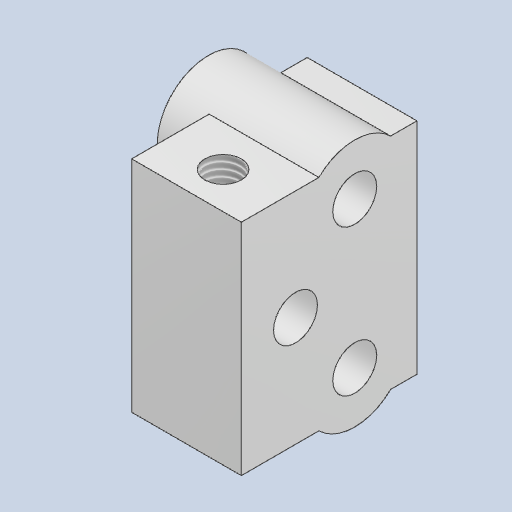
# Autodesk Inventor part: moving_part
Saved by Autodesk Inventor 2024 (Build 280153000, 153)
## iProperties
Created: 2024-09-19
Part Number: moving_part
Material: アルミニウム
Document SubType Name: Modeling
Designer: 1412z
Density: 2.7 g/cm^3
Appearance: サテン
Author: 1412z
Autodesk Inventor part; units mm, degrees
ref_plane "YZ Plane" through (0, 0, 0) normal (1, 0, 0) x (0, 1, 0)
ref_plane "XZ Plane" through (0, 0, 0) normal (0, 1, 0) x (-1, 0, 0)
ref_plane "XY Plane" through (0, 0, 0) normal (0, 0, 1) x (1, 0, 0)
sketch "スケッチ1" plane through (0, 0, 0) normal (1, 0, 0) x (0, 1, 0)
  point P0 (0, 0)
sketch "スケッチ2" plane through (0, 0, 0) normal (0, 0, 1) x (1, 0, 0)
  line L0 (-3.75, 7.5) -> (3.75, 7.5)
  line L1 (3.75, 7.5) -> (3.75, -7.5)
  line L2 (3.75, -7.5) -> (-3.75, -7.5)
  line L3 (-3.75, -7.5) -> (-3.75, 7.5)
  line L4 (-3.75, 7.5) -> (3.75, -7.5) construction
  line L5 (3.75, 7.5) -> (-3.75, -7.5) construction
  point P0 (0, 0)
  dimension "d0" = 7.5
  dimension "d1" = 15
  constraints: 12 end point, 2 midpoint, 2 parallel, 1 horizontal, 1 perpendicular
  measures "d0" distance of L1.end L2.end
  measures "d1" distance of L0.end L1.end
extrude "押し出し1" add sketch "スケッチ2" along normal blind 12
sketch "スケッチ3" plane through (-3.75, 7.5, 0) normal (0, 1, 0) x (1, 0, 0)
  circle A0 centre (3.75, -9.5) radius 1.25
  point P0 (3.75, 0)
  dimension "d4" = 2.5
  constraints: 1 centre point
  measures "d4" diameter of A0
extrude "押し出し2" cut sketch "スケッチ3" against normal blind 6
sketch "スケッチ4" plane through (3.75, -7.5, 0) normal (1, 0, 0) x (0, 0, -1)
  circle A0 centre (-8.3, 7.5) radius 1.5
  point P0 (0, 7.5)
  dimension "d7" = 3
  constraints: 1 centre point
  measures "d7" diameter of A0
extrude "押し出し3" cut sketch "スケッチ4" against normal blind 20
sketch "スケッチ5" plane through (3.75, -7.5, 0) normal (1, 0, 0) x (0, 0, -1)
  circle A0 centre (-4.25, 2.5) radius 1.5
  circle A1 centre (-4.25, 12.5) radius 1.5
  point P0 (0, 7.5)
  dimension "d10" = 3
  dimension "d11" = 3
  constraints: 2 centre point
  measures "d10" diameter of A0
  measures "d11" diameter of A1
extrude "押し出し4" cut sketch "スケッチ5" against normal blind 20
sketch "スケッチ6" plane through (3.75, -7.5, 0) normal (1, 0, 0) x (0, 0, -1)
  circle A0 centre (-4.25, 2.5) radius 1.5 projected
  circle A1 centre (-4.25, 2.5) radius 3.5
  circle A2 centre (-4.25, 12.5) radius 1.5 projected
  circle A3 centre (-4.25, 12.5) radius 3.5
  point P0 (0, 7.5)
  dimension "d14" = 7
  dimension "d15" = 7
  constraints: 2 centre point, 2 coincident
  measures "d14" diameter of A1
  measures "d15" diameter of A3
extrude "押し出し5" add sketch "スケッチ6" against normal blind 10
sketch "スケッチ7" plane through (-3.75, -7.5, 12) normal (0, -1, 0) x (1, 0, 0)
  arc A0 (4.1, -3.7) -> (3.4, -3.7) centre (3.75, -2.5) ccw projected
  circle A1 centre (3.75, -2.5) radius 1.25
  point P0 (3.75, -12)
  constraints: 1 centre point, 1 coincident
extrude "押し出し6" cut sketch "スケッチ7" against normal blind 6
thread "ねじ1" size "M2.5x0.45" class "6H" standard "ANSI Metric M Profile" full length
thread "ねじ2" size "M2.5x0.45" class "6H" standard "ANSI Metric M Profile" full length
